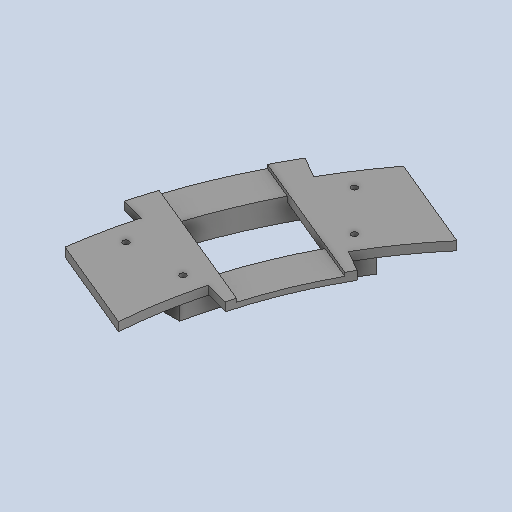
# Autodesk Inventor part: Battery Module Third Iteration Top wING
Saved by Autodesk Inventor 2023 (Build 270158000, 158)
## iProperties
Created: 2023-03-06
Part Number: Battery Module Third Iteration Top wING
Material: PLA Plastic
Document SubType Name: Modeling
Designer: mihal
Density: 1.25002 g/cm^3
Appearance: Generic
Mass: 68.0802 g
Surface Area: 262.43 cm^2
Volume: 54.4631 cm^3
Author: mihal
Autodesk Inventor part; units mm, degrees
ref_plane "YZ Plane" through (0, 0, 0) normal (1, 0, 0) x (0, 1, 0)
sketch "Sketch1" plane through (0, 0, 0) normal (0, 1, 0) x (-1, 0, 0)
  circle A0 centre (0, 0) radius 217.5
  circle A1 centre (0, 0) radius 312.5
  line L0 (0, 0) -> (220.9709, -220.9709)
  line L1 (0, 0) -> (312.5, 0) construction
  line L2 (312.1398, -15) -> (216.9821, -15)
  line L3 (231.3228, -210.1096) -> (164.0361, -142.8229)
  circle A2 centre (0, 0) radius 240
  circle A3 centre (0, 0) radius 290
  line L4 (285.6571, -50) -> (234.7339, -50)
  line L5 (237.3454, -166.6348) -> (201.3373, -130.6266)
  dimension "d0" = 435
  dimension "d1" = 625
  dimension "d2" = 45
  dimension "d3" = 15
  dimension "d4" = 15
  dimension "d5" = 22.5
  dimension "d6" = 22.5
  dimension "d7" = 35
  dimension "d8" = 35
  constraints: 12 end point, 9 point on circle, 4 centre point, 4 coincident, 4 parallel, 1 equal length, 1 horizontal
  measures "d0" diameter of A0
  measures "d1" diameter of A1
  measures "d2" angle of L0 L1
  measures "d3" distance between parallel lines of L2 L1
  measures "d4" distance between parallel lines of L0 L3
  measures "d5" radial gap between concentric circles of A0 A2
  measures "d6" radial gap between concentric circles of A1 A3
  measures "d7" distance between parallel lines of L4 L2
  measures "d8" distance between parallel lines of L3 L5
extrude "Extrusion1" add sketch "Sketch1" along normal blind 10 contours A2 L4 A3 L5
sketch "Sketch2" plane through (0, 10, 0) normal (0, 1, 0) x (1, 0, 0)
  arc A0 (-237.3454, 166.6348) -> (-285.6571, 50) centre (0, 0) ccw projected
  line L0 (-285.6571, 50) -> (-234.7339, 50) projected
  arc A1 (-201.3373, 130.6266) -> (-234.7339, 50) centre (0, 0) ccw projected
  line L1 (-201.3373, 130.6266) -> (-237.3454, 166.6348) projected
  circle A2 centre (0, 0) radius 245
  circle A3 centre (0, 0) radius 285
  line L2 (-279.6426, 55) -> (-238.7467, 55)
  line L3 (-236.6281, 158.8463) -> (-207.7103, 129.9286)
  line L4 (-239.8437, 50) -> (-280.5798, 50)
  line L5 (-204.9504, 134.2398) -> (-233.7552, 163.0445)
  dimension "d11" = 5
  dimension "d12" = 5
  dimension "d13" = 5
  dimension "d14" = 5
  constraints: 8 end point, 8 point on circle, 4 point on line, 2 centre point, 2 coincident, 1 horizontal, 1 parallel
  measures "d11" radial gap between concentric circles of A0 A3
  measures "d12" radial gap between concentric circles of A1 A2
  measures "d13" distance between parallel lines of L1 L3
  measures "d14" distance between parallel lines of L0 L2
extrude "Extrusion2" cut sketch "Sketch2" against normal up to surface (10 mm away) contours L3 A2 L2 A3
sketch "Sketch3" plane through (0, 10, 0) normal (0, 1, 0) x (1, 0, 0)
  arc A0 (-236.6281, 158.8463) -> (-279.6426, 55) centre (0, 0) ccw projected
  line L0 (-236.6281, 158.8463) -> (-207.7103, 129.9286) projected
  arc A1 (-207.7103, 129.9286) -> (-238.7467, 55) centre (0, 0) ccw projected
  line L1 (-238.7467, 55) -> (-279.6426, 55) projected
  arc A2 (-237.3454, 166.6348) -> (-285.6571, 50) centre (0, 0) ccw projected
  line L2 (-285.6571, 50) -> (-234.7339, 50) projected
  arc A3 (-201.3373, 130.6266) -> (-234.7339, 50) centre (0, 0) ccw projected
  line L3 (-201.3373, 130.6266) -> (-237.3454, 166.6348) projected
  circle A4 centre (0, 0) radius 217.5
  circle A5 centre (0, 0) radius 312.5
  line L4 (0, 0) -> (100, 0) construction
  line L5 (0, 0) -> (-220.9709, 220.9709)
  line L6 (0, 0) -> (312.5, 0) construction
  line L7 (-312.1398, 15) -> (-216.9821, 15)
  line L8 (-164.0361, 142.8229) -> (-231.3228, 210.1096)
  line L9 (-437.5, 0) -> (437.5, 0) projected
  dimension "d17" = 435
  dimension "d18" = 625
  dimension "d21" = 135
  dimension "d22" = 15
  dimension "d23" = 15
  constraints: 10 end point, 5 point on circle, 2 centre point, 2 coincident, 2 horizontal, 2 parallel, 1 equal length
  measures "d17" diameter of A4
  measures "d18" diameter of A5
  measures "d21" angle of L6 L5
  measures "d22" distance between parallel lines of L5 L8
  measures "d23" distance between parallel lines of L9 L7
extrude "Extrusion3" add sketch "Sketch3" along normal blind 5 contours L0 A1 L1 A0 | L3 A3 L2 A2 | A4 L7 A5 L8
sketch "Sketch4" plane through (0, 15, 0) normal (0, 1, 0) x (1, 0, 0)
  arc A0 (-231.3228, 210.1096) -> (-312.1398, 15) centre (0, 0) ccw projected
  line L0 (-312.1398, 15) -> (-216.9821, 15) projected
  arc A1 (-164.0361, 142.8229) -> (-216.9821, 15) centre (0, 0) ccw projected
  line L1 (-164.0361, 142.8229) -> (-231.3228, 210.1096) projected
  circle A2 centre (0, 0) radius 217.5
  circle A3 centre (0, 0) radius 312.5
  line L2 (0, 0) -> (4.6194, -1.9134) construction
  line L3 (0, 0) -> (5, 0) construction
  circle A4 centre (4.6194, -1.9134) radius 242.5
  circle A5 centre (4.6194, -1.9134) radius 297.5
  line L4 (0, 0) -> (-288.7124, 119.5886) construction
  line L5 (0, 0) -> (-270.6329, 156.25)
  line L6 (0, 0) -> (-301.8518, 80.881)
  circle A6 centre (4.6194, -1.9134) radius 228.75
  circle A7 centre (4.6194, -1.9134) radius 311.25
  point P0 (-253.3489, 146.271)
  point P1 (-217.3642, 196.151)
  point P2 (-282.5739, 75.7155)
  point P3 (-292.3994, 15)
  point P4 (-205.7173, 118.7709)
  point P5 (-188.3605, 108.75)
  point P6 (-178.396, 157.1828)
  point P7 (-210.0889, 56.2931)
  point P8 (-229.4479, 61.4804)
  point P9 (-237.2901, 15)
  point P10 (-295.8554, 79.2742)
  point P11 (-265.2567, 153.146)
  point P12 (-193.8094, 111.8959)
  point P13 (-216.1663, 57.9216)
  dimension "d26" = 625
  dimension "d27" = 435
  dimension "d28" = 5
  dimension "d29" = 22.5
  dimension "d30" = 485
  dimension "d31" = 595
  dimension "d33" = 15
  dimension "d36" = 457.5
  dimension "d37" = 622.5
  constraints: 10 end point, 6 centre point, 6 coincident, 4 point on circle, 1 concentric, 1 equal length, 1 horizontal, 1 other
  measures "d26" diameter of A3
  measures "d27" diameter of A2
  measures "d28" distance of L2.start L2.end
  measures "d29" angle of L2 L3
  measures "d30" diameter of A4
  measures "d31" diameter of A5
  measures "d33" angle of L0 L6
  measures "d36" diameter of A6
  measures "d37" diameter of A7
extrude "Extrusion4" cut sketch "Sketch4" against normal blind 10 contours L1 A7 L5 A0 | L5 A7 L6 A0 | L1 A5 L5 A7 | L6 A7 L0 A0 | L6 A5 L0 A7 | L1 A6 L5 A4 | L1 A1 L5 A6 | L6 A6 L0 A4 | L5 A1 L6 A6 | L6 A1 L0 A6
sketch "Sketch5" plane through (0, 15, 0) normal (0, 1, 0) x (1, 0, 0)
  arc A0 (-282.5739, 75.7155) -> (-292.3994, 15) centre (4.6194, -1.9134) ccw projected
  line L0 (-292.3994, 15) -> (-237.2901, 15) projected
  arc A1 (-229.4479, 61.4804) -> (-237.2901, 15) centre (4.6194, -1.9134) ccw projected
  line L1 (-229.4479, 61.4804) -> (-216.1663, 57.9216) projected
  arc A2 (-193.8094, 111.8959) -> (-216.1663, 57.9216) centre (4.6194, -1.9134) ccw projected
  line L2 (-193.8094, 111.8959) -> (-205.7173, 118.7709) projected
  arc A3 (-178.396, 157.1828) -> (-205.7173, 118.7709) centre (4.6194, -1.9134) ccw projected
  line L3 (-178.396, 157.1828) -> (-217.3642, 196.151) projected
  arc A4 (-217.3642, 196.151) -> (-253.3489, 146.271) centre (4.6194, -1.9134) ccw projected
  line L4 (-253.3489, 146.271) -> (-265.2567, 153.146) projected
  arc A5 (-265.2567, 153.146) -> (-295.8554, 79.2742) centre (4.6194, -1.9134) ccw projected
  line L5 (-295.8554, 79.2742) -> (-282.5739, 75.7155) projected
  arc A6 (-157.7572, 146.5246) -> (-215.1597, 7.9427) centre (4.6194, -1.9134) ccw
  arc A7 (-254.0861, 186.4253) -> (-311.4886, 47.8434) centre (4.6194, -1.9134) ccw
  line L6 (-311.4886, 47.8434) -> (-215.1597, 7.9427)
  line L7 (-157.7572, 146.5246) -> (-254.0861, 186.4253)
  line L8 (-291.0221, 120.5453) -> (-198.6341, 82.2769) construction
  line L9 (-282.9381, 117.1968) -> (-206.718, 85.6254) construction
  point P0 (0, 0)
  point P1 (-244.8281, 101.4111)
  point P2 (-244.8281, 101.4111)
  point P3 (-232.656, 177.5487)
  point P4 (-179.7358, 155.6284)
  point P5 (-237.1383, 17.0465)
  point P6 (-290.0585, 38.9667)
  dimension "d38" = 150
  dimension "d39" = 104.2656
  constraints: 8 end point, 8 point on circle, 2 centre point, 1 coincident, 1 midpoint
  measures "d38" distance between parallel lines of L6 L7
  measures "d39" distance of L7.start L7.end
extrude "Extrusion5" cut sketch "Sketch5" against normal blind 10 contours L6 A1 L0 A0 | A4 L3 A3 L7
ref_plane "Work Plane2" through (-220.8757, 0, -44.2597) normal (-0.9238795, 0, -0.3826834) x (0, 1, 0)
ref_plane "Work Plane1" through (-234.7339, 0, -50) normal (-0.9238795, 0, -0.3826834) x (0, 1, 0)
sketch "Sketch7" plane through (0, 10, 0) normal (0, -1, 0) x (1, 0, 0)
  arc A0 (-279.6426, -55) -> (-236.6281, -158.8463) centre (0, 0) ccw projected
  line L0 (-236.6281, -158.8463) -> (-207.7103, -129.9286) projected
  arc A1 (-238.7467, -55) -> (-207.7103, -129.9286) centre (0, 0) ccw projected
  arc A2 (-238.7467, -55) -> (-207.7103, -129.9286) centre (0, 0) ccw projected
  line L1 (-238.7467, -55) -> (-279.6426, -55) projected
  arc A3 (-279.6426, -55) -> (-236.6281, -158.8463) centre (0, 0) ccw projected
  arc A4 (-291.5761, -93.715) -> (-272.4419, -139.9089) centre (4.6194, 1.9134) ccw projected
  line L2 (-195.885, -108.198) -> (-272.4419, -139.9089) projected
  arc A5 (-215.0192, -62.0041) -> (-195.885, -108.198) centre (4.6194, 1.9134) ccw projected
  line L3 (-215.0192, -62.0041) -> (-291.5761, -93.715) projected
  arc A6 (-279.6426, -55) -> (-236.6281, -158.8463) centre (0, 0) ccw projected
  line L4 (-279.6426, -55) -> (-238.7467, -55) projected
  arc A7 (-238.7467, -55) -> (-207.7103, -129.9286) centre (0, 0) ccw projected
  line L5 (-207.7103, -129.9286) -> (-236.6281, -158.8463) projected
  arc A8 (-285.6571, -50) -> (-237.3454, -166.6348) centre (0, 0) ccw projected
  line L6 (-201.3373, -130.6266) -> (-237.3454, -166.6348) projected
  arc A9 (-234.7339, -50) -> (-201.3373, -130.6266) centre (0, 0) ccw projected
  line L7 (-285.6571, -50) -> (-234.7339, -50) projected
  line L8 (-233.2223, -155.4405) -> (-236.0507, -152.6121) construction
  line L9 (-236.0507, -152.6121) -> (-238.8791, -155.4405) construction
  line L10 (-209.8621, -132.0804) -> (-212.6905, -129.2519) construction
  line L11 (-212.6905, -129.2519) -> (-209.8621, -126.4235) construction
  circle A10 centre (-212.6905, -129.2519) radius 1.75
  circle A11 centre (-236.0507, -152.6121) radius 1.75
  line L12 (-274.8261, -55) -> (-274.8261, -59) construction
  line L13 (-274.8261, -59) -> (-278.8261, -59) construction
  line L14 (-241.7898, -55) -> (-241.7898, -59) construction
  line L15 (-241.7898, -59) -> (-237.7898, -59) construction
  circle A12 centre (-241.7898, -59) radius 1.75
  circle A13 centre (-274.8261, -59) radius 1.75
  line L16 (-233.2223, -162.5116) -> (-226.8583, -156.1476)
  line L17 (-226.8583, -156.1476) -> (-236.0507, -146.9553)
  line L18 (-236.0507, -146.9553) -> (-242.4147, -153.3192)
  line L19 (-242.4147, -153.3192) -> (-233.2223, -162.5116)
  line L20 (-209.155, -138.4443) -> (-201.3373, -130.6266)
  line L21 (-201.3373, -130.6266) -> (-210.5297, -121.4342)
  line L22 (-210.5297, -121.4342) -> (-218.3474, -129.2519)
  line L23 (-218.3474, -129.2519) -> (-209.155, -138.4443)
  line L24 (-285.6571, -50) -> (-270.8261, -50)
  line L25 (-270.8261, -50) -> (-270.8261, -63)
  line L26 (-270.8261, -63) -> (-285.6571, -63)
  line L27 (-285.6571, -63) -> (-285.6571, -50)
  line L28 (-234.7339, -50) -> (-245.7898, -50)
  line L29 (-245.7898, -50) -> (-245.7898, -63)
  line L30 (-245.7898, -63) -> (-234.7339, -63)
  line L31 (-234.7339, -63) -> (-234.7339, -50)
  line L32 (-236.6281, -158.8463) -> (-207.7103, -129.9286) projected
  line L33 (-238.7467, -55) -> (-279.6426, -55) projected
  arc A14 (-279.6426, -55) -> (-236.6281, -158.8463) centre (0, 0) ccw projected
  line L34 (-236.6281, -158.8463) -> (-207.7103, -129.9286) projected
  arc A15 (-238.7467, -55) -> (-207.7103, -129.9286) centre (0, 0) ccw projected
  line L35 (-238.7467, -55) -> (-279.6426, -55) projected
  point P0 (-214.4385, -125.3431)
  point P1 (-277.9496, -63)
  point P2 (-270.8261, -55)
  point P3 (-236.7615, -63)
  point P4 (-245.7898, -55)
  point P5 (-212.6905, -134.9088)
  point P6 (-211.9634, -122.8679)
  point P7 (-241.0878, -151.9923)
  point P8 (-230.3939, -152.6121)
  dimension "d51" = 4
  dimension "d52" = 4
  dimension "d54" = 4
  dimension "d55" = 4
  dimension "d56" = 3.5
  dimension "d57" = 3.5
  dimension "d58" = 4
  dimension "d59" = 4
  dimension "d60" = 4
  dimension "d61" = 4
  dimension "d62" = 3.5
  dimension "d63" = 3.5
  dimension "d64" = 4
  dimension "d65" = 4
  dimension "d66" = 5
  dimension "d71" = 4
  dimension "d72" = 4
  dimension "d73" = 4
  dimension "d74" = 4
  dimension "d75" = 4
  dimension "d76" = 4
  constraints: 48 end point, 11 perpendicular, 11 point on line, 8 parallel, 4 centre point, 4 coincident, 4 point on circle, 1 collinear, 1 midpoint
  measures "d51" distance of L8.start L8.end
  measures "d52" distance of L8.end L9.end
  measures "d54" distance of L10.start L10.end
  measures "d55" distance of L10.end L11.end
  measures "d56" diameter of A10
  measures "d57" diameter of A11
  measures "d58" distance of L12.start L12.end
  measures "d59" distance of L12.end L13.end
  measures "d60" distance of L14.start L14.end
  measures "d61" distance of L14.end L15.end
  measures "d62" diameter of A12
  measures "d63" diameter of A13
  measures "d64" distance from line of L17 L8.end
  measures "d65" distance from line of L18 L8.end
  measures "d66" distance from line of L19 L8.end
  measures "d71" distance from line of L23 L10.end
  measures "d72" distance from line of L22 L10.end
  measures "d73" distance from line of L25 A13.centre
  measures "d74" distance from line of L26 A13.centre
  measures "d75" distance from line of L29 L14.end
  measures "d76" distance from line of L30 L14.end
extrude "Extrusion7" add sketch "Sketch7" along normal blind 10 contours L1 L25 L26 A0 | L1 A1 L30 L29 | L18 L17 L0 A0 | A1 L0 L23 L22
extrude "Extrusion8" cut sketch "Sketch7" against normal up to next contours A10 | A11 | A12 | A13
ref_plane "Work Plane4" through (-216.1663, 15, -57.9216) normal (0.9238795, 0, 0.3826834) x (0, -1, 0)
sketch "Sketch9" plane through (-216.1663, 15, -57.9216) normal (0.9238795, 0, 0.3826834) x (0, -1, 0)
  line L0 (5, 58.4214) -> (5, 0) projected
  line L1 (0, 58.4214) -> (5, 58.4214) projected
  line L2 (0, 0) -> (0, 58.4214) projected
  line L3 (0, 0) -> (5, 0) projected
  line L4 (15, -14.4241) -> (15, 72.8455) projected
  line L5 (15, 72.8455) -> (5, 72.8455) projected
  line L6 (5, -14.4241) -> (5, 72.8455) projected
  line L7 (15, -14.4241) -> (5, -14.4241) projected
  line L8 (-2, 5.2107) -> (2, 5.2107)
  line L9 (2, 5.2107) -> (2, 53.2107)
  line L10 (2, 53.2107) -> (-2, 53.2107)
  line L11 (-2, 53.2107) -> (-2, 5.2107)
  line L12 (-2, 5.2107) -> (2, 53.2107) construction
  line L13 (2, 5.2107) -> (-2, 53.2107) construction
  point P0 (15, 29.2107)
  point P1 (0, 29.2107)
  dimension "d85" = 4
  dimension "d86" = 48
  constraints: 12 end point, 3 midpoint, 2 parallel, 1 horizontal, 1 perpendicular
  measures "d85" distance of L10.end L9.end
  measures "d86" distance of L9.end L8.end
extrude "Extrusion10" cut sketch "Sketch9" against normal up to next contours L10 L9 L8 L2 | L2 L8 L11 L10
sketch "Sketch10" plane through (0, 10, 0) normal (0, -1, 0) x (1, 0, 0)
  arc A0 (-291.2664, -94.6691) -> (-272.8976, -139.0153) centre (4.6194, 1.9134) ccw projected
  line L0 (-214.736, -62.9692) -> (-291.2664, -94.6691) projected
  arc A1 (-214.736, -62.9692) -> (-196.3672, -107.3154) centre (4.6194, 1.9134) ccw projected
  line L1 (-196.3672, -107.3154) -> (-272.8976, -139.0153) projected
  line L2 (-245.7898, -63) -> (-245.7898, -55) projected
  line L3 (-245.7898, -55) -> (-270.8261, -55) projected
  line L4 (-270.8261, -55) -> (-270.8261, -63) projected
  line L5 (-270.8261, -63) -> (-277.9496, -63) projected
  arc A2 (-277.9496, -63) -> (-241.0878, -151.9923) centre (0, 0) ccw projected
  line L6 (-241.0878, -151.9923) -> (-236.0507, -146.9553) projected
  line L7 (-236.0507, -146.9553) -> (-230.3939, -152.6121) projected
  line L8 (-230.3939, -152.6121) -> (-212.6905, -134.9088) projected
  line L9 (-212.6905, -134.9088) -> (-218.3474, -129.2519) projected
  line L10 (-218.3474, -129.2519) -> (-211.9634, -122.8679) projected
  arc A3 (-236.7615, -63) -> (-211.9634, -122.8679) centre (0, 0) ccw projected
  line L11 (-236.7615, -63) -> (-245.7898, -63) projected
  point P0 (-216.0774, -115.4796)
  point P1 (-234.4462, -71.1334)
  point P2 (-271.5548, -86.5043)
  point P3 (-253.186, -130.8505)
extrude "Extrusion11" cut sketch "Sketch10" against normal blind 10 contours L0 A3 L1 A2
body "Solid1"
